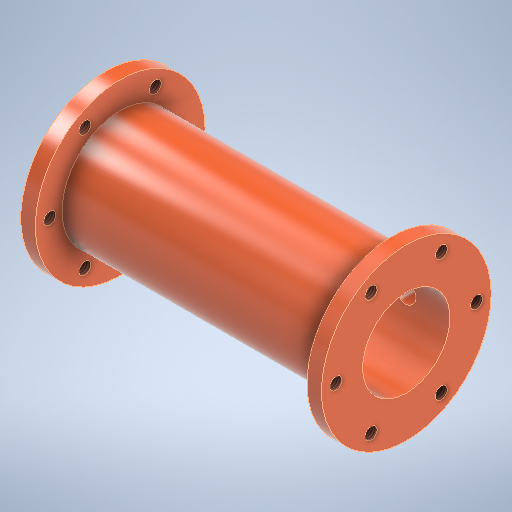
# Autodesk Inventor part: 154
Saved by Autodesk Inventor 2025.1 (Build 291241000, 241)
## iProperties
Created: 2024-08-01
Part Number: 154
Material: Stainless Steel
Document SubType Name: Modeling
Designer: ffogue
Density: 8 g/cm^3
Appearance: Smooth - Light Orange
Author: ffogue
Autodesk Inventor part; units mm, degrees
ref_plane "YZ Plane" through (0, 0, 0) normal (1, 0, 0) x (0, 1, 0)
sketch "Sketch1" plane through (0, 0, 0) normal (0, 0, 1) x (1, 0, 0)
  line L0 (-31, 0) -> (-31, 17.5)
  line L1 (-31, 17.5) -> (-28, 17.5)
  line L2 (-28, 17.5) -> (-28, 12)
  line L3 (-28, 12) -> (28, 12)
  line L4 (28, 12) -> (28, 17.5)
  line L5 (28, 17.5) -> (31, 17.5)
  line L6 (31, 17.5) -> (31, 0)
  line L7 (31, 0) -> (-31, 0)
  point P0 (0, 0)
  point P1 (0, 0)
  dimension "d0" = 24
  dimension "d1" = 35
  dimension "d2" = 3
  dimension "d3" = 3
  dimension "d4" = 56
  constraints: 16 end point, 6 perpendicular, 2 point on line, 1 coincident, 1 midpoint, 1 vertical
  measures "d0" diameter of L3 L7
  measures "d1" diameter of L1 L7
  measures "d2" distance of L0.end L1.end
  measures "d3" distance of L4.end L5.end
  measures "d4" distance of L2.end L3.end
revolve "Revolution1" add sketch "Sketch1" angle 360 about axis through (31, 0, 0) along (-1, 0, 0)
sketch "Sketch2" plane through (31, 0, 0) normal (1, 0, 0) x (0, 0, -1)
  circle A0 centre (0, 0) radius 17.5 projected
  point P0 (0, 0)
  constraints: 1 coincident
hole "Hole1" at (31, 0, 0) direction (-1, 0, 0) diameter 18 end through all
ref_plane "Work Plane1" through (31, 0, 0) normal (1, 0, 0) x (0, 0, -1)
sketch "Sketch3" plane through (31, 0, 0) normal (1, 0, 0) x (0, 0, -1)
  line L0 (0, 0) -> (-20.6833, 0) construction
  line L1 (0, 0) -> (-12.5574, -7.25) construction
  circle A0 centre (0, 0) radius 14.5 construction
  dimension "d15" = 29
  dimension "d14" = 30
  constraints: 4 end point, 2 coincident, 1 horizontal, 3 other
  measures "d14" angle of L0 L1
hole "Hole2" at (31, -7.25, 12.5574) direction (-1, 0, 0) diameter 2.459 depth 3 thread size "M3x0.5" class "6H" standard "ISO Metric profile"
pattern_circular "Circular Pattern1" count 6 over 360 about axis through (29.5, 0, 0) along (-1, 0, 0) of "Hole2"
mirror "Mirror1" about plane through (0, 0, 0) normal (1, 0, 0) of "Hole2", "Circular Pattern1"
ref_plane "Work Plane3" through (0, 12, 0) normal (0, 1, 0) x (-1, 0, 0)
sketch "Sketch5" plane through (0, 12, 0) normal (0, 1, 0) x (-1, 0, 0)
  line L0 (28, -17.5) -> (28, 17.5) projected
  line L1 (-28, -17.5) -> (-28, 17.5) projected
  point P0 (0, 0)
  point P1 (22, 0)
  point P2 (-22, 0)
  dimension "d37" = 6
  dimension "d38" = 6
  constraints: 2 horizontal alignment
  measures "d37" distance from line of L0 point (22, 0)
  measures "d38" distance from line of L1 point (-22, 0)
hole "Hole4" at (-22, 12, 0) at (22, 12, 0) direction (0, -1, 0) diameter 4 depth 3.5
body "Solid1"
